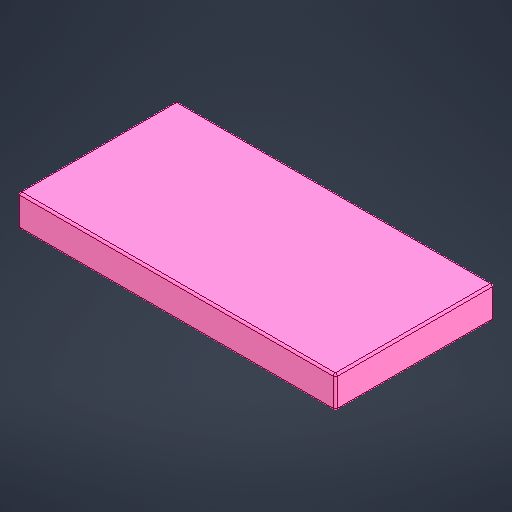
# Autodesk Inventor part: plate
Saved by Autodesk Inventor 2026 (Build 300175000, 175)
## iProperties
Created: 2025-04-21
Part Number: plate
Material: Generic
Document SubType Name: Modeling
Designer: Paul Juschitz
Density: 1 g/cm^3
Appearance: Pink
Author: Paul Juschitz
Autodesk Inventor part; units mm, degrees
ref_plane "YZ Plane" through (0, 0, 0) normal (1, 0, 0) x (0, 1, 0)
ref_plane "XZ Plane" through (0, 0, 0) normal (0, 1, 0) x (-1, 0, 0)
ref_plane "XY Plane" through (0, 0, 0) normal (0, 0, 1) x (1, 0, 0)
sketch "Sketch1" plane through (0, 0, 0) normal (0, 1, 0) x (-1, 0, 0)
  line L0 (40, 20) -> (-40, 20)
  line L1 (-40, 20) -> (-40, -20)
  line L2 (-40, -20) -> (40, -20)
  line L3 (40, -20) -> (40, 20)
  line L4 (40, 20) -> (-40, -20) construction
  line L5 (-40, 20) -> (40, -20) construction
  point P0 (0, 0)
  dimension "d0" = 80
  dimension "d1" = 40
  constraints: 12 end point, 2 midpoint, 2 parallel, 1 horizontal, 1 perpendicular
  measures "d0" distance of L1.end L2.end
  measures "d1" distance of L0.end L1.end
extrude "Extrusion1" add sketch "Sketch1" along normal blind 8
shell "Shell1" thickness 1.6 removed faces 1 at (13.3333, 0, 6.6667)
fillet "Fillet1" radius 0.5 20 edges at (0, 8, 20) (-40, 8, 0) (-40, 4, 20) (-40, 0, 0) (0, 0, 20) (40, 4, 20) (-40, 4, -20) (0, 0, -20) (0, 8, -20) (40, 4, -20) (40, 8, 0) (38.4, 0, 0) (40, 0, 0) (0, 0, 18.4) (0, 0, -18.4) (-38.4, 0, 0) (38.4, 6.4, 0) (0, 6.4, -18.4) (0, 6.4, 18.4) (-38.4, 6.4, 0)
sketch "Sketch4" plane through (-37.9, 6.4, 17.9) normal (0, -1, 0) x (1, 0, 0)
  circle A0 centre (36.9, -25.855) radius 1.5
  circle A1 centre (24, -25.855) radius 1.5
  circle A2 centre (24, -9.945) radius 1.5
  circle A3 centre (36.9, -9.945) radius 1.5
  line L0 (0, -35.8) -> (0, 0) projected
  line L1 (0, -17.9) -> (71.9831, -17.9)
  line L2 (36.9, -9.945) -> (24, -25.855) construction
  line L3 (24, -9.945) -> (36.9, -25.855) construction
  line L4 (40.9, -5.945) -> (20, -5.945)
  line L5 (20, -5.945) -> (20, -29.855)
  line L6 (20, -29.855) -> (40.9, -29.855)
  line L7 (40.9, -29.855) -> (40.9, -5.945)
  line L8 (40.9, -5.945) -> (20, -29.855) construction
  line L9 (20, -5.945) -> (40.9, -29.855) construction
  point P0 (30.45, -17.9)
  dimension "d24" = 3
  dimension "d25" = 3
  dimension "d28" = 15.91
  dimension "d29" = 12.9
  dimension "d30" = 4
  dimension "d31" = 4
  dimension "d32" = 20
  constraints: 18 end point, 4 centre point, 4 midpoint, 2 equal radius, 2 horizontal, 2 horizontal alignment, 2 parallel, 2 vertical alignment, 1 perpendicular, 1 symmetric about line
  measures "d24" diameter of A0
  measures "d25" diameter of A1
  measures "d28" distance of L2.end L3.start
  measures "d29" distance of L2.start L3.start
  measures "d30" distance from line of L4 L3.start
  measures "d31" distance from line of L5 L3.start
  measures "d32" distance between parallel lines of L0 L5
extrude "Extrusion4" add sketch "Sketch4" along normal blind 4
equation "\"d0\" = plate_depth"
equation "\"d1\" = plate_width"
equation "\"plate_width\" = 40"
equation "\"plate_depth\" = 80"
body "Solid1"
